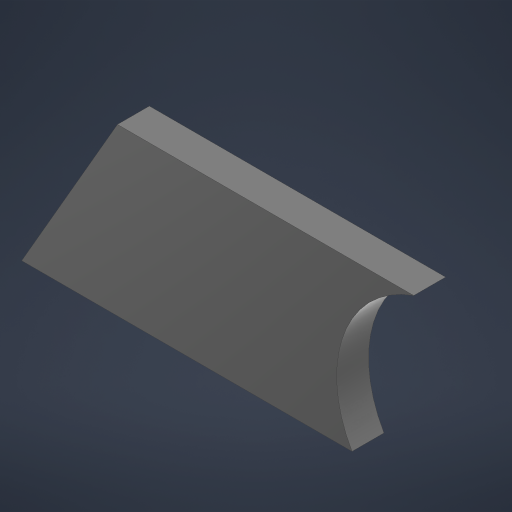
# Autodesk Inventor part: bok_lewy
Saved by Autodesk Inventor 2024 (Build 280153000, 153)
## iProperties
Created: 2024-05-25
Part Number: bok_lewy
Material: ABS Plastic
Document SubType Name: Modeling
Designer: Adam
Density: 1.06 g/cm^3
Appearance: Smooth - White
Mass: 4.70038 g
Surface Area: 30.9781 cm^2
Volume: 4.70038 cm^3
Author: Adam
Autodesk Inventor part; units mm, degrees
ref_plane "YZ Plane" through (0, 0, 0) normal (1, 0, 0) x (0, 1, 0)
ref_plane "XZ Plane" through (0, 0, 0) normal (0, 1, 0) x (-1, 0, 0)
ref_plane "XY Plane" through (0, 0, 0) normal (0, 0, 1) x (1, 0, 0)
sketch "Sketch1" plane through (0, 0, 0) normal (0, 0, 1) x (1, 0, 0)
  line L0 (15.0111, 26) -> (0, 0)
  arc A0 (61.4575, 26) -> (51.7851, 0) centre (67.3735, 9) ccw
  line L1 (61.4575, 26) -> (15.0111, 26)
  line L2 (0, 0) -> (51.7851, 0)
  dimension "d0" = 18
  dimension "d25" = 26
  constraints: 6 end point, 2 point on circle, 1 centre point, 1 coincident, 1 parallel
  measures "d0" radius of A0
  measures "d25" distance between parallel lines of L1 L2
extrude "Extrusion1" add sketch "Sketch1" along normal blind 5
sketch "Sketch2" plane through (0, 0, 0) normal (0, -1, 0) x (1, 0, 0)
  circle A0 centre (40.7851, -3) radius 1.55
  line L0 (0, 0) -> (51.7851, 0) projected
  line L1 (44.7851, 0) -> (36.7851, 0)
  line L2 (36.7851, 0) -> (36.7851, -7)
  line L3 (36.7851, -7) -> (44.7851, -7)
  line L4 (44.7851, -7) -> (44.7851, 0)
  line L5 (15, 0) -> (7, 0)
  line L6 (0, 0) -> (0, 5) projected
  line L7 (51.7851, 0) -> (51.7851, 5) projected
  point P0 (40.7851, 0)
  point P1 (44.7851, -3.5)
  point P2 (15, -3.5)
  point P3 (36.7851, 0)
  dimension "d3" = 3.1
  dimension "d5" = 8
  dimension "d6" = 7
  dimension "d9" = 3
  dimension "d17" = 4
  dimension "d27" = 7
  constraints: 10 end point, 2 horizontal, 2 midpoint, 2 parallel, 2 point on line, 1 centre point, 1 perpendicular
  measures "d3" diameter of A0
  measures "d5" distance of L3.end L2.end
  measures "d6" distance of L2.end L1.end
  measures "d9" distance of point (40.785, 0) A0.centre
  measures "d17" distance from line of A0.centre L4
  measures "d27" distance between parallel lines of L4 L7
extrude "Extrusion2" add sketch "Sketch2" against normal blind 3
sketch "Sketch3" plane through (0, 3, 0) normal (0, 1, 0) x (1, 0, 0)
  line L0 (42.2876, 5.6024) -> (43.7901, 3)
  line L1 (43.7901, 3) -> (42.2876, 0.3976)
  line L2 (42.2876, 0.3976) -> (39.2826, 0.3976)
  line L3 (39.2826, 0.3976) -> (37.7801, 3)
  line L4 (37.7801, 3) -> (39.2826, 5.6024)
  line L5 (39.2826, 5.6024) -> (42.2876, 5.6024)
  circle A0 centre (40.7851, 3) radius 1.55 projected
  line L6 (61.4575, 0) -> (15.0111, 0) projected
  point P0 (0, 0)
  point P1 (42.3218, 4.7299)
  dimension "d15" = 6.01
  constraints: 12 end point, 2 coincident, 1 parallel, 13 other
  measures "d15" distance of L0.start L2.end
fillet "Fillet1" radius 4 2 edges at (44.7851, 1.5, -7) (36.7851, 1.5, -7)
fillet "Fillet2" radius 1 3 edges at (40.7851, 3, 0) (44.7851, 1.5, 0) (36.7851, 1.5, 0)
extrude "Extrusion3" cut sketch "Sketch3" along normal blind 3 and the other way blind 2
chamfer "Chamfer1" distance 0.2 angle 45 8 edges at (40.7851, 3.2018, -0.3976) (38.3574, 3, -2) (39.1182, 3.0518, -0.6823) (43.2127, 3, -2) (42.452, 3.0518, -0.6823) (43.0388, 3, -4.3012) (38.5313, 3, -4.3012) (40.7851, 3, -5.6024)
body "Solid1"
